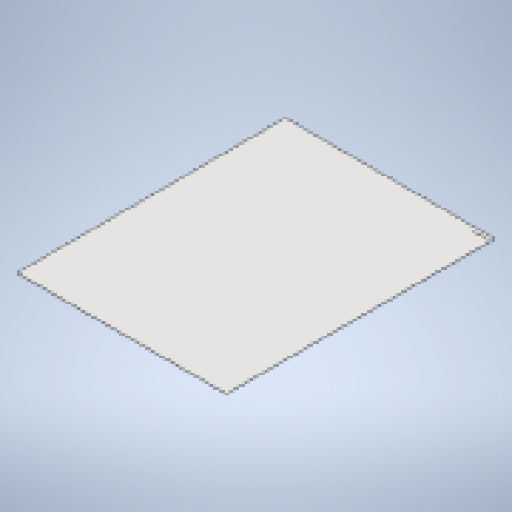
# Autodesk Inventor part: BSH 045 back
Saved by Autodesk Inventor 2025 (Build 290162010, 162A)
## iProperties
Created: 2024-07-23
Part Number: BSH 045 back
Material: 09g2s
Document SubType Name: Sheet Metal
Designer: admin
Mass: 66048.3 g
Surface Area: 56294.5 cm^2
Volume: 8413.8 cm^3
Density: 7.85 g/cm^3
Sheet Metal Rule: AISI304 3mm Die 32
Sheet Metal Width: 1479,000 mm
Sheet Metal Length: 1895,000 mm
Sheet Metal Area: 2802705,000 mm^2
Appearance: Default
Flat Pattern Width: 147.9 cm
Flat Pattern Length: 189.5 cm
Flat Pattern Area: 28027 cm^2
Stock Number: БШК 045 борт
Author: admin
Autodesk Inventor part; units mm, degrees
ref_plane "YZ Plane" through (0, 0, 0) normal (1, 0, 0) x (0, 1, 0)
ref_plane "XZ Plane" through (0, 0, 0) normal (0, 1, 0) x (-1, 0, 0)
ref_plane "XY Plane" through (0, 0, 0) normal (0, 0, 1) x (1, 0, 0)
sketch "Sketch6" plane through (0, 0, 0) normal (0, 0, 1) x (1, 0, 0)
  line L0 (739.5, 947.5) -> (-739.5, 947.5)
  line L1 (-739.5, 947.5) -> (-739.5, -947.5)
  line L2 (-739.5, -947.5) -> (739.5, -947.5)
  line L3 (739.5, -947.5) -> (739.5, 947.5)
  line L4 (739.5, 947.5) -> (-739.5, -947.5) construction
  line L5 (-739.5, 947.5) -> (739.5, -947.5) construction
  point P0 (0, 0)
  dimension "d40" = 1479
  dimension "d41" = 1895
  measures "d40" distance of L2.end L1.end
  measures "d41" distance of L1.end L0.end
extrude "Plate5" add sketch "Sketch6" along normal blind 3
sketch "Sketch7" plane through (0, 0, 0) normal (0, 0, -1) x (-1, 0, 0)
  line L0 (-714.5, 922.5) -> (-514.5, 922.5) construction
  line L1 (-514.5, 922.5) -> (-514.5, 907.5) construction
  line L2 (-514.5, 907.5) -> (-714.5, 907.5) construction
  line L3 (-714.5, 907.5) -> (-714.5, 922.5) construction
  line L4 (-739.5, 947.5) -> (739.5, 947.5) projected
  line L5 (-739.5, -947.5) -> (-739.5, 947.5) projected
  point P0 (0, 0)
  dimension "d43" = 200
  dimension "d44" = 15
  dimension "d45" = 25
  dimension "d46" = 25
  constraints: 2 parallel, 2 other
  measures "d43" distance of L3.end L0.end
  measures "d44" distance between parallel lines of L0 L2
  measures "d45" distance between parallel lines of L4 L0
  measures "d46" distance between parallel lines of L5 L3
mark "Mark1"
equation "\"d42\" = Thickness"
equation "\"BendReliefWidth\" = Thickness"
equation "\"BendReliefDepth\" = 0.5 * Thickness"
equation "\"CornerReliefSize\" = 4 * Thickness"
equation "\"MinimumRemnant\" = 2 * Thickness"
equation "\"TransitionRadius\" = BendRadius"
equation "\"JacobiRadiusSize\" = BendRadius"
equation "\"GapSize\" = Thickness"
equation "\"Thickness\" = 3"
equation "\"BendRadius\" = 5"
body "Solid4"
